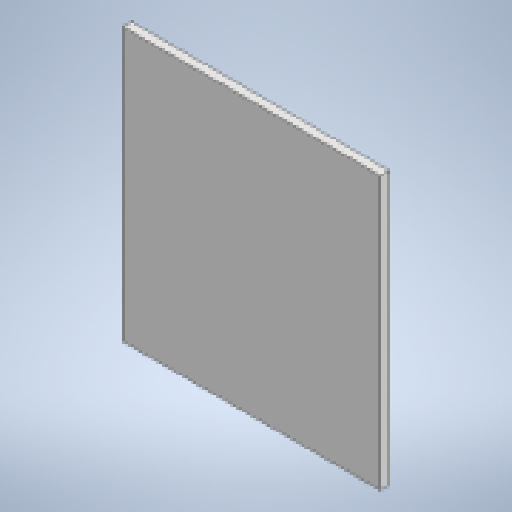
# Autodesk Inventor part: pcb
Saved by Autodesk Inventor 2023 (Build 270158000, 158)
## iProperties
Created: 2023-12-19
Part Number: pcb
Material: Ogólny
Document SubType Name: Modeling
Designer: Kamil
Density: 1 g/cm^3
Appearance: Domyślna
Author: Kamil
Autodesk Inventor part; units mm, degrees
ref_plane "YZ Plane" through (0, 0, 0) normal (1, 0, 0) x (0, 1, 0)
ref_plane "XZ Plane" through (0, 0, 0) normal (0, 1, 0) x (-1, 0, 0)
ref_plane "XY Plane" through (0, 0, 0) normal (0, 0, 1) x (1, 0, 0)
sketch "Szkic1" plane through (0, 0, 0) normal (0, 0, 1) x (1, 0, 0)
  line L0 (-43, 25) -> (-7, 25) projected
  line L1 (-7, 25) -> (-7, 11) projected
  line L2 (-7, 11) -> (7, 11) projected
  line L3 (7, 11) -> (7, -11) projected
  line L4 (7, -11) -> (-7, -11) projected
  line L5 (-7, -11) -> (-7, -25) projected
  line L6 (-7, -25) -> (-43, -25) projected
  line L7 (-7, -11) -> (7, -11)
  line L8 (7, -11) -> (7, -25)
  line L9 (7, -25) -> (-7, -25)
  line L10 (-7, -25) -> (-7, -11)
  line L11 (-7, 11) -> (7, 11)
  line L12 (7, 11) -> (7, 25)
  line L13 (7, 25) -> (-7, 25)
  line L14 (-7, 25) -> (-7, 11)
  line L15 (-43, -25) -> (-43, 25) projected
  point P0 (0, 0)
  point P1 (7, 11)
  point P2 (7, 11)
  constraints: 16 end point, 4 parallel, 2 horizontal, 2 perpendicular, 1 point on line
extrude "Wyciągnięcie proste1" add sketch "Szkic1" along normal blind 1.6
ref_plane "Płaszczyzna konstrukcyjna1" through (-17.9997, 25, -4.7) normal (0, 1, 0) x (0, 0, 1)
sketch "Szkic3" plane through (0, 0, 1.6) normal (0, 0, 1) x (1, 0, 0)
  line L0 (-43, -25) -> (7, -25) projected
  line L1 (7, -25) -> (7, 25) projected
  line L2 (7, 25) -> (-43, 25) projected
  line L3 (-13, -25) -> (-9, -25)
  line L4 (-9, -25) -> (-9, -17)
  line L5 (-9, -17) -> (-13, -17)
  line L6 (-13, -17) -> (-13, -25)
  line L7 (7, 25) -> (-40.2936, 25) projected
  line L8 (-9, 25) -> (-13, 25)
  line L9 (-13, 25) -> (-13, 17)
  line L10 (-13, 17) -> (-9, 17)
  line L11 (-9, 17) -> (-9, 25)
  line L12 (-43, 25) -> (-43, -25) projected
  point P0 (0, 0)
  point P1 (-35.2314, 25)
  point P2 (-35.7424, 25)
  point P3 (-11, 25)
  dimension "d4" = 16
  dimension "d5" = 16
  dimension "d6" = 8
  dimension "d7" = 8
  dimension "d8" = 4
  dimension "d9" = 4
  constraints: 16 end point, 4 parallel, 2 horizontal, 2 perpendicular, 2 point on line, 1 midpoint
  measures "d4" distance between parallel lines of L1 L4
  measures "d5" distance between parallel lines of L1 L11
  measures "d6" distance between parallel lines of L5 L0
  measures "d7" distance from line of point (-11, 25) L10
  measures "d8" distance between parallel lines of L6 L4
  measures "d9" distance between parallel lines of L9 L11
extrude "Wyciągnięcie proste3" cut sketch "Szkic3" against normal through all contours L6 L5 L4 L0 | L2 L11 L10 L9
sketch "Szkic4" plane through (-40.2936, 25, 1.6) normal (0, 1, 0) x (1, 0, 0)
  line L0 (4.9241, -3) -> (-0.6358, 17.75) projected
  line L1 (-0.6358, 17.75) -> (-2.7064, 17.75) projected
  line L2 (-2.7064, 17.75) -> (2.8536, -3) projected
  line L3 (2.8536, -3) -> (4.9241, -3) projected
  line L4 (27.2936, 0) -> (27.2936, 1.6) projected
  line L5 (47.2936, 1.6) -> (31.2936, 1.6) projected
  line L6 (27.2936, 0) -> (-2.7064, 0) projected
  line L7 (27.2936, 1.6) -> (-2.7064, 1.6) projected
  line L8 (-2.7064, 1.6) -> (-2.7064, 0) projected
  line L9 (31.2936, 1.6) -> (31.2936, 0) projected
  line L10 (47.2936, 0) -> (31.2936, 0) projected
  line L11 (47.2936, 1.6) -> (47.2936, 0) projected
  point P0 (40.2936, 1.6)
  point P1 (3.6916, 1.6)
  point P2 (4.1203, 0)
extrude "Wyciągnięcie proste4" cut sketch "Szkic4" against normal through all contours L6 L2 L7 L0 | L6 L8 L7 L2
